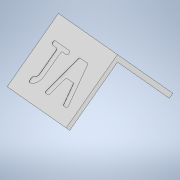
# Autodesk Inventor part: TableroEscritoSimplificado
Saved by Autodesk Inventor 2022 (Build 260153000, 153)
## iProperties
Created: 2022-08-28
Part Number: TableroEscritoSimplificado
Material: Generic
Document SubType Name: Modeling
Designer: Usuario
Density: 1 g/cm^3
Appearance: Default
Author: Usuario
Autodesk Inventor part; units mm, degrees
ref_plane "YZ Plane" through (0, 0, 0) normal (1, 0, 0) x (0, 1, 0)
ref_plane "XZ Plane" through (0, 0, 0) normal (0, 1, 0) x (-1, 0, 0)
ref_plane "XY Plane" through (0, 0, 0) normal (0, 0, 1) x (1, 0, 0)
sketch "Sketch1" plane through (0, 0, 0) normal (0, 1, 0) x (-1, 0, 0)
  line L0 (17, 250) -> (0, 250)
  line L1 (0, 250) -> (0, 0)
  line L2 (0, 0) -> (17, 0)
  line L3 (17, 0) -> (17, 250)
  line L4 (17, 0) -> (-233, 0)
  line L5 (-233, 0) -> (-233, -17)
  line L6 (-233, -17) -> (17, -17)
  line L7 (17, -17) -> (17, 0)
  dimension "d0" = 17
  dimension "d1" = 250
  dimension "d2" = 250
  constraints: 16 end point, 4 parallel, 3 perpendicular, 2 horizontal
  measures "d0" distance of L6.end L2.end
  measures "d1" distance of L2.end L0.start
  measures "d2" distance of L5.end L6.end
extrude "Extrusion1" add sketch "Sketch1" along normal blind 284.5
sketch "Sketch2" plane through (233, 0, -17) normal (0, 0, -1) x (-1, 0, 0)
  line L0 (0, 0) -> (250, 0) projected
  line L1 (250, 0) -> (250, 284.5) projected
  line L2 (0, 284.5) -> (250, 284.5) projected
  line L3 (0, 0) -> (0, 284.5) projected
  line L4 (182.1785, 237.4156) -> (168.1785, 237.4156)
  line L5 (168.1785, 237.4156) -> (168.1785, 159.4156)
  line L6 (168.1785, 159.4156) -> (182.1785, 159.4156)
  line L7 (182.1785, 159.4156) -> (182.1785, 237.4156)
  line L8 (168.1785, 208.4156) -> (82.1785, 208.4156)
  line L9 (82.1785, 208.4156) -> (82.1785, 188.4156)
  line L10 (82.1785, 188.4156) -> (168.1785, 188.4156)
  line L11 (168.1785, 188.4156) -> (168.1785, 208.4156)
  arc A0 (64.6656, 225.9286) -> (82.1785, 208.4156) centre (82.1785, 225.9286) ccw
  line L12 (82.1785, 225.9286) -> (64.6656, 225.9286) construction
  line L13 (82.1785, 225.9286) -> (82.1785, 208.4156) construction
  arc A1 (44.6656, 225.9286) -> (82.1785, 188.4156) centre (82.1785, 225.9286) ccw
  line L14 (64.6656, 225.9286) -> (44.6656, 225.9286)
  line L15 (182.3419, 116.525) -> (46.5005, 150.394)
  line L16 (46.5005, 150.394) -> (46.5005, 130.394)
  line L17 (46.5005, 130.394) -> (114.6042, 113.4139)
  line L18 (114.6042, 113.4139) -> (114.6042, 93.4139)
  line L19 (182.3419, 116.525) -> (182.3419, 95.525)
  line L20 (133.1096, 95.525) -> (42.0362, 95.525)
  line L21 (182.3419, 74.525) -> (46.5005, 40.6559)
  line L22 (46.5005, 40.6559) -> (46.5005, 60.6559)
  line L23 (46.5005, 60.6559) -> (114.6042, 77.6361)
  line L24 (114.6042, 77.6361) -> (114.6042, 97.6361)
  line L25 (182.3419, 74.525) -> (182.3419, 95.525)
  point P0 (233, 0)
  dimension "d5" = 90
  dimension "d6" = 21
  dimension "d7" = 140
  dimension "d8" = 20
  dimension "d9" = 20
  dimension "d12" = 68.1037
  dimension "d13" = 78
  dimension "d14" = 20
  dimension "d15" = 29
  dimension "d16" = 14
  dimension "d18" = 86
  dimension "d20" = 76
  constraints: 44 end point, 5 parallel, 5 symmetric about line, 4 horizontal, 4 point on circle, 3 vertical, 2 centre point, 2 perpendicular, 1 coincident, 1 point on line
  measures "d5" angle of L12 L13
  measures "d6" distance of L15.start L19.end
  measures "d7" distance of L15.start L15.end
  measures "d8" distance of L15.end L16.end
  measures "d9" distance of L17.end L18.end
  measures "d12" horizontal distance of L16.end L17.end
  measures "d13" distance of L6.end L4.start
  measures "d14" distance of L8.end L9.end
  measures "d15" distance between parallel lines of L6 L10
  measures "d16" distance of L4.start L4.end
  measures "d18" distance of L8.start L8.end
  measures "d20" angle of L16 L15
extrude "Extrusion2" cut sketch "Sketch2" against normal blind 1 contours L7 L6 L5 L4 | L5 L10 L9 L8 | L9 A1 L14 A0 | L19 L25 L21 L22 L23 L24 L18 L17 L16 L15
fillet "Fillet1" radius 5 16 edges at (50.6581, 116.525, -16.5) (50.6581, 74.525, -16.5) (50.8215, 159.4156, -16.5) (64.8215, 188.4156, -16.5) (118.3958, 113.4139, -16.5) (118.3958, 77.6361, -16.5) (186.4995, 40.6559, -16.5) (186.4995, 60.6559, -16.5) (186.4995, 130.394, -16.5) (186.4995, 150.394, -16.5) (168.3344, 225.9286, -16.5) (188.3344, 225.9286, -16.5) (64.8215, 237.4156, -16.5) (50.8215, 237.4156, -16.5) (64.8215, 159.4156, -16.5) (64.8215, 208.4156, -16.5)
equation "\"d15\" = 0.5 * d13 - 0.5 * d14"
body "Solid1"
